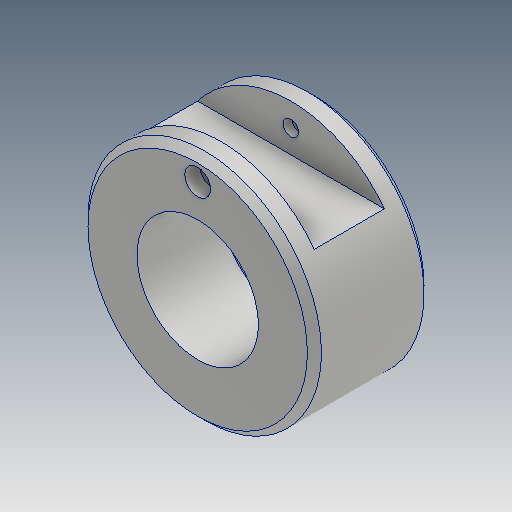
# Autodesk Inventor part: 200-30-ROCKER-BOGIE-BEARING-01
Saved by Autodesk Inventor 2018.2 (Build 222227000, 227)
## iProperties
Manager: feesmrt
Company: FRANC0R
Created: 2017-11-20
Part Number: 200-30-ROCKER-BOGIE-BEARING-01
Material: Aluminium 6061
Document SubType Name: Modeling
Designer: feesmrt
Density: 2.7 g/cm^3
Appearance: Aluminium - flach
Project: Rescue Robot
Cost Center: -
Description: Bogie Bearing Housing and Connector
Engineer: feesmrt
Authority: feesmrt
Stock Number: 200-30-ROCKER-BOGIE-BEARING-01
Author: feesmrt
Title: Bogie Bearing Housing and Connector
Subject: Rescue Robot
Revision Number: 1
Autodesk Inventor part; units mm, degrees
ref_plane "YZ Plane" through (0, 0, 0) normal (1, 0, 0) x (0, 1, 0)
ref_plane "XZ Plane" through (0, 0, 0) normal (0, 1, 0) x (-1, 0, 0)
ref_plane "XY Plane" through (0, 0, 0) normal (0, 0, 1) x (1, 0, 0)
sketch "Skizze3" plane through (0, 0, 0) normal (1, 0, 0) x (0, 1, 0)
  line L0 (0, 60) -> (0, -10) construction
  line L1 (-35, 0) -> (35, 0) construction
  line L2 (25, 0) -> (25, 22.5) construction
  line L3 (25, 50) -> (-25, 50)
  line L4 (-25, 50) -> (-25, 26)
  line L5 (11.1, 0) -> (11.1, 26) construction
  line L6 (11.1, 26) -> (-11.1, 26) construction
  line L7 (-11.1, 26) -> (-11.1, 0) construction
  line L8 (11.1, 22.5) -> (25, 22.5)
  line L9 (11.1, 22.5) -> (11.1, 26)
  line L10 (11.1, 26) -> (-25, 26)
  line L11 (-25, 26) -> (-25, 0) construction
  line L12 (25, 22.5) -> (25, 50)
  point P0 (0, 0)
  dimension "d8" = 100
  dimension "d9" = 50
  dimension "d10" = 52
  dimension "d11" = 22.2
  dimension "d13" = 45
  constraints: 22 end point, 8 perpendicular, 6 point on line, 3 vertical, 1 collinear, 2 other
  measures "d8" diameter of L3 L1
  measures "d9" distance between parallel lines of L2 L4
  measures "d10" diameter of L6 L1
  measures "d11" distance between parallel lines of L7 L5
  measures "d13" diameter of L8 L1
revolve "Grundkörper" add sketch "Skizze3" angle 360 about axis through (0, 0, 0) along (0, 1, 0)
sketch "Skizze4" plane through (0, 0, 0) normal (1, 0, 0) x (0, 1, 0)
  line L0 (-25, 50) -> (25, 50) construction
  line L1 (0, 48) -> (0, -8) construction
  line L2 (-15, 50) -> (-15, 30)
  line L3 (-15, 30) -> (15, 30)
  line L4 (15, 30) -> (15, 50)
  line L5 (-15, 50) -> (15, 50)
  point P0 (0, 0)
  dimension "d17" = 30
  dimension "d18" = 20
  constraints: 8 end point, 2 perpendicular, 2 point on line, 1 collinear, 1 vertical, 1 other
  measures "d17" distance between parallel lines of L4 L2
  measures "d18" distance between parallel lines of L0 L3
extrude "Profil_Ausschnitt" cut sketch "Skizze4" along normal through all both and the other way through all
sketch "Skizze5" plane through (0, -25, 0) normal (0, -1, 0) x (1, 0, 0)
  circle A0 centre (0, 0) radius 50 construction
  line L0 (0, 70) -> (0, -70) construction
  line L1 (-40, 30) -> (40, 30) construction
  line L2 (0, 30) -> (0, 50) construction
  point P0 (0, 40)
  constraints: 2 end point, 2 midpoint, 1 point on circle, 1 point on line
hole "ISO4762_M6_Boh" at (0, -25, 40) direction (0, 1, 0) diameter 6.6 end up to face face through (-3.0733, 15, 40.9552) facing (0, -1, 0) counterbore diameter 11 counterbore depth 6.4
mirror "Spiegelung_ISO4762_M6_Boh" about plane through (0, 0, 0) normal (0, 1, 0) of "ISO4762_M6_Boh"
chamfer "Fase1" distance 3 angle 45 2 edges at (0, -25, -50) (0, 25, -50)
